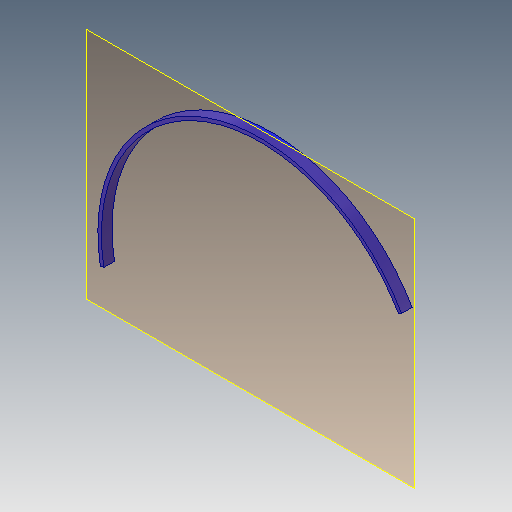
# Autodesk Inventor part: FleLG
Saved by Autodesk Inventor 2019.4 (Build 234330000, 330)
## iProperties
Created: 2019-06-16
Part Number: FleLG
Material: PVC、軟質
Document SubType Name: Modeling
Designer: AzLIer
Density: 1.3 g/cm^3
Appearance: 青 - 壁塗料 - 光沢
Mass: 18.1676 g
Surface Area: 113.307 cm^2
Volume: 13.9751 cm^3
Author: AzLIer
Autodesk Inventor part; units mm, degrees
ref_plane "YZ Plane" through (0, 0, 0) normal (1, 0, 0) x (0, 1, 0)
ref_plane "XZ Plane" through (0, 0, 0) normal (0, 1, 0) x (-1, 0, 0)
ref_plane "XY Plane" through (0, 0, 0) normal (0, 0, 1) x (1, 0, 0)
ref_plane "作業平面1" through (0, 0, 0) normal (0, 0, 1) x (1, 0, 0)
sketch "スケッチ1" plane through (0, 0, 0) normal (0, 0, 1) x (1, 0, 0)
  arc A0 (140.8609, 25) -> (-136.764, -76.0472) centre (10.9571, -50) ccw projected
  arc A1 (143.7188, 26.65) -> (-140.0139, -76.6203) centre (10.9571, -50) ccw
  line L0 (143.7188, 26.65) -> (140.8609, 25)
  line L1 (-140.0139, -76.6203) -> (-136.764, -76.0472)
  point P0 (0, 0)
  dimension "d0" = 3.3
  constraints: 4 end point, 2 line through centre, 2 point on circle, 1 centre point
  measures "d0" radial gap between concentric circles of A0 A1
extrude "押し出し1" add sketch "スケッチ1" against normal blind 10
